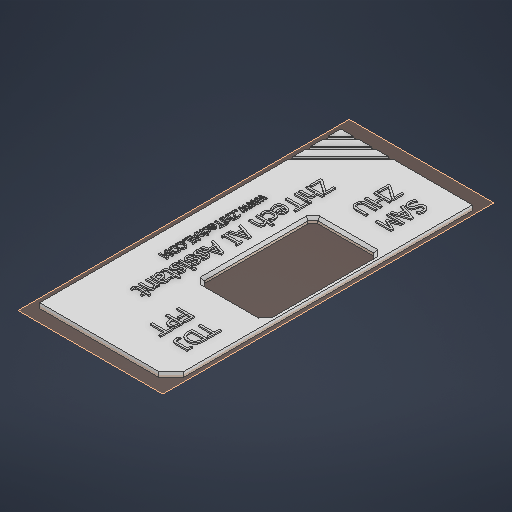
# Autodesk Inventor part: Part6
Saved by Autodesk Inventor 2026 (Build 300175000, 175)
## iProperties
Created: 2025-06-06
Part Number: Part6
Material: Generic
Document SubType Name: Sheet Metal
Designer: ziyuz
Density: 1 g/cm^3
Sheet Metal Rule: Default_mm
Appearance: Default
Author: ziyuz
Autodesk Inventor part; units mm, degrees
(part 1 of 2)
ref_plane "YZ Plane" through (0, 0, 0) normal (1, 0, 0) x (0, 1, 0)
ref_plane "XZ Plane" through (0, 0, 0) normal (0, 1, 0) x (-1, 0, 0)
ref_plane "XY Plane" through (0, 0, 0) normal (0, 0, 1) x (1, 0, 0)
sketch "Sketch1" plane through (0, 0, 0) normal (0, 1, 0) x (-1, 0, 0)
  line L0 (-29.0932, -58.6501) -> (-29.0932, -48.6501)
  line L1 (-29.0932, -58.6501) -> (-29.0932, 55.3499)
  line L2 (-29.0932, 55.3499) -> (-24.0932, 60.3499)
  line L3 (-29.0932, 55.3499) -> (-24.0932, 60.3499)
  line L4 (-24.0932, 60.3499) -> (22.9068, 60.3499)
  line L5 (-24.0932, 60.3499) -> (22.9068, 60.3499)
  line L6 (22.9068, 60.3499) -> (22.9068, -58.6501)
  line L7 (22.9068, -58.6501) -> (-29.0932, -58.6501)
  line L8 (-29.0932, -38.6501) -> (0.9068, -38.6501)
  line L9 (-29.0932, -38.6501) -> (2.9068, -38.6501)
  line L10 (2.9068, -38.6501) -> (2.9068, 31.3499)
  line L11 (2.9068, 31.3499) -> (-29.0932, 31.3499)
  line L12 (-29.0932, -38.6501) -> (-29.0932, -23.6501)
  line L13 (-29.0932, -23.6501) -> (2.9068, -23.6501)
  line L14 (-29.0932, 31.3499) -> (-29.0932, 21.3499)
  line L15 (-29.0932, 21.3499) -> (2.9068, 21.3499)
  line L16 (-29.0932, -23.6501) -> (-29.0932, 21.3499)
  line L17 (-29.0932, -23.6501) -> (-27.0932, -23.6501)
  line L18 (-27.0932, -23.6501) -> (-27.0932, 21.3499)
  line L19 (-29.0932, 21.3499) -> (-27.0932, 21.3499)
  line L20 (0.9068, -38.6501) -> (0.9068, 31.3499)
  line L21 (0.9068, -23.6501) -> (-1.0932, -23.6501)
  line L22 (-1.0932, -23.6501) -> (-1.0932, 21.3499)
  point P0 (0, 0)
  point P1 (-27.0932, 58.3499)
  dimension "d0" = 32
  dimension "d1" = 70
  dimension "d2" = 15
  dimension "d3" = 10
  dimension "d4" = 2
  dimension "d5" = 2
  constraints: 46 end point, 11 point on line, 8 perpendicular, 5 collinear, 1 vertical
  measures "d0" distance of L8.start L9.end
  measures "d1" distance of L9.end L10.end
  measures "d2" distance of L8.start L12.end
  measures "d3" distance of L11.end L14.end
  measures "d4" distance of L12.end L17.end
  measures "d5" distance of L21.start L21.end
extrude "Extrusion1" add sketch "Sketch1" along normal blind 2 contours L0 L1 L8 L9 L10 L11 L2 L4 L6 L7 | L1 L13 L20 L8 | L1 L15 L18 L13 | L20 L13 L10 L9 | L1 L11 L20 L15 | L20 L15 L10 L13 | L13 L22 L15 L20 | L20 L11 L10 L15
chamfer "Chamfer1" distance 2 angle 45 4 edges at (27.0932, 1, 21.3499) (27.0932, 1, -23.6501) (1.0932, 1, -23.6501) (1.0932, 1, 21.3499)
ref_plane "Work Plane1" through (0, 1, 0) normal (0, 1, 0) x (1, 0, 0)
sketch "Sketch7" plane through (0, 2, 0) normal (0, 1, 0) x (1, 0, 0)
  line L0 (22.864, -34.3556) -> (22.864, -48.4389) construction
  line L1 (22.864, -48.4389) -> (6.7205, -48.4389) construction
  line L2 (6.7205, -48.4389) -> (6.7205, -34.3556) construction
  line L3 (6.7205, -34.3556) -> (22.864, -34.3556) construction
  line L4 (22.2427, 49.0186) -> (22.2427, 34.9352) construction
  line L5 (22.2427, 34.9352) -> (6.0992, 34.9352) construction
  line L6 (6.0992, 34.9352) -> (6.0992, 49.0186) construction
  line L7 (6.0992, 49.0186) -> (22.2427, 49.0186) construction
  line L8 (-2.8839, 40.5637) -> (-2.8839, -41.6354) construction
  line L9 (-2.8839, -41.6354) -> (-17.8366, -41.6354) construction
  line L10 (-17.8366, -41.6354) -> (-17.8366, 40.5637) construction
  line L11 (-17.8366, 40.5637) -> (-2.8839, 40.5637) construction
  line L12 (16.764, -36.3971) -> (22.1423, -36.3971)
  line L13 (22.1423, -36.3971) -> (22.1423, -34.3506)
  line L14 (22.1423, -34.3506) -> (22.864, -34.3506)
  line L15 (22.864, -34.3506) -> (22.864, -39.2543)
  line L16 (22.864, -39.2543) -> (22.1423, -39.2543)
  line L17 (22.1423, -39.2543) -> (22.1423, -37.2078)
  line L18 (22.1423, -37.2078) -> (16.764, -37.2078)
  line L19 (16.764, -37.2078) -> (16.764, -36.3971)
  spline S0 degree 2 poles (19.8091, -44.6821) (18.9737, -44.6821) (17.6291, -44.0048) (17.2534, -43.4363) knots 0 0 0 1 2 2 2
  spline S1 degree 2 poles (17.2534, -43.4363) (16.9617, -42.9717) (16.764, -42.0176) (16.764, -41.2761) knots 0 0 0 1 2 2 2
  line L20 (16.764, -41.2761) -> (16.764, -39.8722)
  line L21 (16.764, -39.8722) -> (22.864, -39.8722)
  line L22 (22.864, -39.8722) -> (22.864, -41.2613)
  spline S2 degree 2 poles (22.864, -41.2613) (22.864, -42.1214) (22.607, -43.1002) (22.3796, -43.4462) knots 0 0 0 1 2 2 2
  spline S3 degree 2 poles (22.3796, -43.4462) (21.989, -44.0345) (20.6989, -44.6821) (19.8091, -44.6821) knots 0 0 0 1 2 2 2
  spline S4 degree 2 poles (19.819, -43.8368) (20.5209, -43.8368) (21.5145, -43.3721) (21.7963, -42.9124) knots 0 0 0 1 2 2 2
  spline S5 degree 2 poles (21.7963, -42.9124) (21.989, -42.5861) (22.1621, -41.8496) (22.1621, -41.3009) knots 0 0 0 1 2 2 2
  line L23 (22.1621, -41.3009) -> (22.1621, -40.6829)
  line L24 (22.1621, -40.6829) -> (17.466, -40.6829)
  line L25 (17.466, -40.6829) -> (17.466, -41.3009)
  spline S6 degree 2 poles (17.466, -41.3009) (17.466, -41.8397) (17.639, -42.6553) (17.8713, -42.9865) knots 0 0 0 1 2 2 2
  spline S7 degree 2 poles (17.8713, -42.9865) (18.158, -43.4116) (19.1071, -43.8368) (19.819, -43.8368) knots 0 0 0 1 2 2 2
  spline S8 degree 2 poles (18.3508, -47.8606) (17.55, -47.8606) (16.68, -46.8818) (16.68, -46.0563) knots 0 0 0 1 2 2 2
  spline S9 degree 2 poles (16.68, -46.0563) (16.68, -45.8586) (16.7492, -45.2011) (16.7986, -44.9787) knots 0 0 0 1 2 2 2
  line L26 (16.7986, -44.9787) -> (17.5796, -44.9787)
  line L27 (17.5796, -44.9787) -> (17.5796, -45.0231)
  spline S10 degree 2 poles (17.5796, -45.0231) (17.5203, -45.1912) (17.3819, -45.6905) (17.3819, -45.9475) knots 0 0 0 1 2 2 2
  spline S11 degree 2 poles (17.3819, -45.9475) (17.3819, -46.3232) (17.5549, -46.7731) (17.7131, -46.8769) knots 0 0 0 1 2 2 2
  spline S12 degree 2 poles (17.7131, -46.8769) (17.8762, -46.9906) (18.3508, -47.0499) (18.6622, -47.0499) knots 0 0 0 1 2 2 2
  line L28 (18.6622, -47.0499) -> (22.2164, -47.0499)
  line L29 (22.2164, -47.0499) -> (22.2164, -45.7597)
  line L30 (22.2164, -45.7597) -> (22.864, -45.7597)
  line L31 (22.864, -45.7597) -> (22.864, -47.8606)
  line L32 (22.864, -47.8606) -> (18.3508, -47.8606)
  line L33 (12.0988, -38.6216) -> (12.0988, -35.7842)
  line L34 (12.0988, -35.7842) -> (10.3785, -35.7842)
  line L35 (10.3785, -35.7842) -> (10.3785, -38.503)
  line L36 (10.3785, -38.503) -> (9.6568, -38.503)
  line L37 (9.6568, -38.503) -> (9.6568, -35.7842)
  line L38 (9.6568, -35.7842) -> (6.7205, -35.7842)
  line L39 (6.7205, -35.7842) -> (6.7205, -34.9735)
  line L40 (6.7205, -34.9735) -> (12.8205, -34.9735)
  line L41 (12.8205, -34.9735) -> (12.8205, -38.6216)
  line L42 (12.8205, -38.6216) -> (12.0988, -38.6216)
  spline S13 degree 2 poles (10.9816, -43.204) (10.5862, -43.204) (9.8743, -42.9222) (9.6272, -42.6701) knots 0 0 0 1 2 2 2
  spline S14 degree 2 poles (9.6272, -42.6701) (9.3157, -42.3538) (8.9944, -41.4986) (8.9944, -40.8461) knots 0 0 0 1 2 2 2
  line L43 (8.9944, -40.8461) -> (8.9944, -40.159)
  line L44 (8.9944, -40.159) -> (6.7205, -40.159)
  line L45 (6.7205, -40.159) -> (6.7205, -39.3483)
  line L46 (6.7205, -39.3483) -> (12.8205, -39.3483)
  line L47 (12.8205, -39.3483) -> (12.8205, -40.8807)
  spline S15 degree 2 poles (12.8205, -40.8807) (12.8205, -41.4244) (12.6426, -42.1857) (12.4399, -42.4774) knots 0 0 0 1 2 2 2
  spline S16 degree 2 poles (12.4399, -42.4774) (12.2076, -42.8184) (11.4908, -43.204) (10.9816, -43.204) knots 0 0 0 1 2 2 2
  spline S17 degree 2 poles (10.9569, -42.3587) (11.2733, -42.3587) (11.7379, -42.1412) (11.8862, -41.9188) knots 0 0 0 1 2 2 2
  spline S18 degree 2 poles (11.8862, -41.9188) (12.0148, -41.726) (12.1186, -41.2119) (12.1186, -40.8312) knots 0 0 0 1 2 2 2
  line L48 (12.1186, -40.8312) -> (12.1186, -40.159)
  line L49 (12.1186, -40.159) -> (9.6865, -40.159)
  line L50 (9.6865, -40.159) -> (9.6865, -40.7126)
  spline S19 degree 2 poles (9.6865, -40.7126) (9.6865, -41.2069) (9.8447, -41.815) (10.0523, -42.0127) knots 0 0 0 1 2 2 2
  spline S20 degree 2 poles (10.0523, -42.0127) (10.2352, -42.1956) (10.6653, -42.3587) (10.9569, -42.3587) knots 0 0 0 1 2 2 2
  line L51 (6.7205, -45.3988) -> (12.0988, -45.3988)
  line L52 (12.0988, -45.3988) -> (12.0988, -43.3523)
  line L53 (12.0988, -43.3523) -> (12.8205, -43.3523)
  line L54 (12.8205, -43.3523) -> (12.8205, -48.256)
  line L55 (12.8205, -48.256) -> (12.0988, -48.256)
  line L56 (12.0988, -48.256) -> (12.0988, -46.2095)
  line L57 (12.0988, -46.2095) -> (6.7205, -46.2095)
  line L58 (6.7205, -46.2095) -> (6.7205, -45.3988)
  point P0 (0, 0)
  constraints: 6 other
extrude "Extrusion6" add sketch "Sketch7" along normal blind 0.5
sketch "Sketch8" plane through (0, 2, 0) normal (0, 1, 0) x (1, 0, 0)
  line L0 (22.2544, 48.9464) -> (22.2544, 32.777) construction
  line L1 (22.2544, 32.777) -> (5.8736, 32.777) construction
  line L2 (5.8736, 32.777) -> (5.8736, 48.9464) construction
  line L3 (5.8736, 48.9464) -> (22.2544, 48.9464) construction
  spline S0 degree 2 poles (15.9369, 46.628) (15.9369, 47.2904) (16.2137, 48.2197) (16.4114, 48.63) knots 0 0 0 1 2 2 2
  line L4 (16.4114, 48.63) -> (17.4297, 48.63)
  line L5 (17.4297, 48.63) -> (17.4297, 48.5707)
  spline S1 degree 2 poles (17.4297, 48.5707) (17.054, 48.1703) (16.6388, 47.1569) (16.6388, 46.6873) knots 0 0 0 1 2 2 2
  spline S2 degree 2 poles (16.6388, 46.6873) (16.6388, 46.015) (17.1974, 45.3279) (17.6571, 45.3279) knots 0 0 0 1 2 2 2
  spline S3 degree 2 poles (17.6571, 45.3279) (18.0229, 45.3279) (18.4777, 45.6888) (18.5914, 46.0793) knots 0 0 0 1 2 2 2
  spline S4 degree 2 poles (18.5914, 46.0793) (18.6705, 46.3611) (18.7792, 46.8307) (18.8682, 47.1817) knots 0 0 0 1 2 2 2
  spline S5 degree 2 poles (18.8682, 47.1817) (18.9523, 47.498) (19.2044, 47.9973) (19.407, 48.1901) knots 0 0 0 1 2 2 2
  spline S6 degree 2 poles (19.407, 48.1901) (19.6097, 48.3779) (20.1535, 48.5856) (20.5094, 48.5856) knots 0 0 0 1 2 2 2
  spline S7 degree 2 poles (20.5094, 48.5856) (21.2509, 48.5856) (22.2544, 47.4288) (22.2544, 46.5341) knots 0 0 0 1 2 2 2
  spline S8 degree 2 poles (22.2544, 46.5341) (22.2544, 46.02) (22.0517, 45.1104) (21.8589, 44.7199) knots 0 0 0 1 2 2 2
  line L6 (21.8589, 44.7199) -> (20.89, 44.7199)
  line L7 (20.89, 44.7199) -> (20.89, 44.7792)
  spline S9 degree 2 poles (20.89, 44.7792) (21.157, 45.0709) (21.5524, 45.9804) (21.5524, 46.4797) knots 0 0 0 1 2 2 2
  spline S10 degree 2 poles (21.5524, 46.4797) (21.5524, 47.0433) (21.0235, 47.7403) (20.5934, 47.7403) knots 0 0 0 1 2 2 2
  spline S11 degree 2 poles (20.5934, 47.7403) (20.2079, 47.7403) (19.7481, 47.33) (19.6443, 46.9444) knots 0 0 0 1 2 2 2
  spline S12 degree 2 poles (19.6443, 46.9444) (19.5751, 46.6873) (19.3972, 45.9409) (19.323, 45.6937) knots 0 0 0 1 2 2 2
  spline S13 degree 2 poles (19.323, 45.6937) (19.1302, 45.0659) (18.3541, 44.4826) (17.7856, 44.4826) knots 0 0 0 1 2 2 2
  spline S14 degree 2 poles (17.7856, 44.4826) (17.4248, 44.4826) (16.7327, 44.7743) (16.4905, 45.0363) knots 0 0 0 1 2 2 2
  spline S15 degree 2 poles (16.4905, 45.0363) (16.2236, 45.3279) (15.9369, 46.0694) (15.9369, 46.628) knots 0 0 0 1 2 2 2
  line L8 (16.0456, 44.3146) -> (22.1456, 42.2582)
  line L9 (22.1456, 42.2582) -> (22.1456, 41.2596)
  line L10 (22.1456, 41.2596) -> (16.0456, 39.2032)
  line L11 (16.0456, 39.2032) -> (16.0456, 40.0584)
  line L12 (16.0456, 40.0584) -> (17.751, 40.6121)
  line L13 (17.751, 40.6121) -> (17.751, 42.9403)
  line L14 (17.751, 42.9403) -> (16.0456, 43.494)
  line L15 (16.0456, 43.494) -> (16.0456, 44.3146)
  line L16 (18.4431, 40.8345) -> (21.3151, 41.7787)
  line L17 (21.3151, 41.7787) -> (18.4431, 42.7179)
  line L18 (18.4431, 42.7179) -> (18.4431, 40.8345)
  line L19 (16.0456, 33.3949) -> (16.0456, 34.2056)
  line L20 (16.0456, 34.2056) -> (21.3003, 34.2056)
  line L21 (21.3003, 34.2056) -> (17.7263, 35.7973)
  line L22 (17.7263, 35.7973) -> (17.7263, 36.2916)
  line L23 (17.7263, 36.2916) -> (21.3003, 37.8685)
  line L24 (21.3003, 37.8685) -> (16.0456, 37.8685)
  line L25 (16.0456, 37.8685) -> (16.0456, 38.6249)
  line L26 (16.0456, 38.6249) -> (22.1456, 38.6249)
  line L27 (22.1456, 38.6249) -> (22.1456, 37.5176)
  line L28 (22.1456, 37.5176) -> (18.7496, 35.995)
  line L29 (18.7496, 35.995) -> (22.1456, 34.5219)
  line L30 (22.1456, 34.5219) -> (22.1456, 33.3949)
  line L31 (22.1456, 33.3949) -> (16.0456, 33.3949)
  line L32 (6.0021, 44.4381) -> (6.0021, 48.6992)
  line L33 (6.0021, 48.6992) -> (6.7584, 48.6992)
  line L34 (6.7584, 48.6992) -> (11.3804, 45.4367)
  line L35 (11.3804, 45.4367) -> (11.3804, 48.5509)
  line L36 (11.3804, 48.5509) -> (12.1021, 48.5509)
  line L37 (12.1021, 48.5509) -> (12.1021, 44.5222)
  line L38 (12.1021, 44.5222) -> (11.3705, 44.5222)
  line L39 (11.3705, 44.5222) -> (6.7238, 47.8193)
  line L40 (6.7238, 47.8193) -> (6.7238, 44.4381)
  line L41 (6.7238, 44.4381) -> (6.0021, 44.4381)
  line L42 (6.0021, 39.2082) -> (6.0021, 40.0189)
  line L43 (6.0021, 40.0189) -> (8.9879, 40.0189)
  line L44 (8.9879, 40.0189) -> (8.9879, 42.8266)
  line L45 (8.9879, 42.8266) -> (6.0021, 42.8266)
  line L46 (6.0021, 42.8266) -> (6.0021, 43.6373)
  line L47 (6.0021, 43.6373) -> (12.1021, 43.6373)
  line L48 (12.1021, 43.6373) -> (12.1021, 42.8266)
  line L49 (12.1021, 42.8266) -> (9.7096, 42.8266)
  line L50 (9.7096, 42.8266) -> (9.7096, 40.0189)
  line L51 (9.7096, 40.0189) -> (12.1021, 40.0189)
  line L52 (12.1021, 40.0189) -> (12.1021, 39.2082)
  line L53 (12.1021, 39.2082) -> (6.0021, 39.2082)
  spline S16 degree 2 poles (5.8736, 35.8418) (5.8736, 36.3806) (6.1554, 37.1814) (6.4371, 37.4632) knots 0 0 0 1 2 2 2
  spline S17 degree 2 poles (6.4371, 37.4632) (6.7535, 37.7845) (7.6433, 38.0465) (8.2958, 38.0465) knots 0 0 0 1 2 2 2
  line L54 (8.2958, 38.0465) -> (12.1021, 38.0465)
  line L55 (12.1021, 38.0465) -> (12.1021, 37.2358)
  line L56 (12.1021, 37.2358) -> (8.2958, 37.2358)
  spline S18 degree 2 poles (8.2958, 37.2358) (7.8707, 37.2358) (7.2973, 37.127) (7.0649, 36.9738) knots 0 0 0 1 2 2 2
  spline S19 degree 2 poles (7.0649, 36.9738) (6.8178, 36.8107) (6.5657, 36.2471) (6.5657, 35.8418) knots 0 0 0 1 2 2 2
  spline S20 degree 2 poles (6.5657, 35.8418) (6.5657, 35.4612) (6.8178, 34.868) (7.0649, 34.7048) knots 0 0 0 1 2 2 2
  spline S21 degree 2 poles (7.0649, 34.7048) (7.2973, 34.5516) (7.8657, 34.4428) (8.276, 34.4428) knots 0 0 0 1 2 2 2
  line L57 (8.276, 34.4428) -> (12.1021, 34.4428)
  line L58 (12.1021, 34.4428) -> (12.1021, 33.6321)
  line L59 (12.1021, 33.6321) -> (8.2958, 33.6321)
  spline S22 degree 2 poles (8.2958, 33.6321) (7.6581, 33.6321) (6.7486, 33.8892) (6.4371, 34.2155) knots 0 0 0 1 2 2 2
  spline S23 degree 2 poles (6.4371, 34.2155) (6.1504, 34.5071) (5.8736, 35.2783) (5.8736, 35.8418) knots 0 0 0 1 2 2 2
  point P0 (0, 0)
  constraints: 2 other
extrude "Extrusion7" add sketch "Sketch8" along normal blind 0.5
sketch "Sketch9" plane through (0, 2, 0) normal (0, 1, 0) x (1, 0, 0)
  line L0 (-3.0335, 37.4291) -> (-3.0335, -37.9904) construction
  line L1 (-3.0335, -37.9904) -> (-36.9755, -37.9904) construction
  line L2 (-36.9755, -37.9904) -> (-36.9755, 37.4291) construction
  line L3 (-36.9755, 37.4291) -> (-3.0335, 37.4291) construction
  line L4 (-9.4054, 32.9209) -> (-9.4054, 37.182)
  line L5 (-9.4054, 37.182) -> (-8.6491, 37.182)
  line L6 (-8.6491, 37.182) -> (-4.0271, 33.9194)
  line L7 (-4.0271, 33.9194) -> (-4.0271, 37.0337)
  line L8 (-4.0271, 37.0337) -> (-3.3054, 37.0337)
  line L9 (-3.3054, 37.0337) -> (-3.3054, 33.0049)
  line L10 (-3.3054, 33.0049) -> (-4.037, 33.0049)
  line L11 (-4.037, 33.0049) -> (-8.6837, 36.3021)
  line L12 (-8.6837, 36.3021) -> (-8.6837, 32.9209)
  line L13 (-8.6837, 32.9209) -> (-9.4054, 32.9209)
  line L14 (-9.4054, 28.5856) -> (-9.4054, 29.3568)
  line L15 (-9.4054, 29.3568) -> (-6.7954, 29.3568)
  spline S0 degree 2 poles (-6.7954, 29.3568) (-6.479, 29.3568) (-5.9352, 29.4161) (-5.7721, 29.5051) knots 0 0 0 1 2 2 2
  spline S1 degree 2 poles (-5.7721, 29.5051) (-5.5991, 29.599) (-5.431, 29.9351) (-5.431, 30.2218) knots 0 0 0 1 2 2 2
  spline S2 degree 2 poles (-5.431, 30.2218) (-5.431, 30.5086) (-5.7375, 31.1166) (-5.9847, 31.4082) knots 0 0 0 1 2 2 2
  line L16 (-5.9847, 31.4082) -> (-9.4054, 31.4082)
  line L17 (-9.4054, 31.4082) -> (-9.4054, 32.1794)
  line L18 (-9.4054, 32.1794) -> (-3.0335, 32.1794)
  line L19 (-3.0335, 32.1794) -> (-3.0335, 31.4082)
  line L20 (-3.0335, 31.4082) -> (-5.3371, 31.4082)
  spline S3 degree 2 poles (-5.3371, 31.4082) (-5.0257, 31.0622) (-4.6994, 30.3949) (-4.6994, 30.0192) knots 0 0 0 1 2 2 2
  spline S4 degree 2 poles (-4.6994, 30.0192) (-4.6994, 29.3469) (-5.5892, 28.5856) (-6.4345, 28.5856) knots 0 0 0 1 2 2 2
  line L21 (-6.4345, 28.5856) -> (-9.4054, 28.5856)
  line L22 (-9.4054, 26.7171) -> (-9.4054, 27.4882)
  line L23 (-9.4054, 27.4882) -> (-4.8279, 27.4882)
  line L24 (-4.8279, 27.4882) -> (-4.8279, 26.7171)
  line L25 (-4.8279, 26.7171) -> (-9.4054, 26.7171)
  line L26 (-4.0667, 26.6627) -> (-4.0667, 27.5377)
  line L27 (-4.0667, 27.5377) -> (-3.2659, 27.5377)
  line L28 (-3.2659, 27.5377) -> (-3.2659, 26.6627)
  line L29 (-3.2659, 26.6627) -> (-4.0667, 26.6627)
  line L30 (-9.4054, 24.1021) -> (-4.0271, 24.1021)
  line L31 (-4.0271, 24.1021) -> (-4.0271, 26.1486)
  line L32 (-4.0271, 26.1486) -> (-3.3054, 26.1486)
  line L33 (-3.3054, 26.1486) -> (-3.3054, 21.2449)
  line L34 (-3.3054, 21.2449) -> (-4.0271, 21.2449)
  line L35 (-4.0271, 21.2449) -> (-4.0271, 23.2914)
  line L36 (-4.0271, 23.2914) -> (-9.4054, 23.2914)
  line L37 (-9.4054, 23.2914) -> (-9.4054, 24.1021)
  spline S5 degree 2 poles (-9.5092, 18.6991) (-9.5092, 19.7965) (-8.2783, 21.0026) (-7.1414, 21.0026) knots 0 0 0 1 2 2 2
  spline S6 degree 2 poles (-7.1414, 21.0026) (-6.0242, 21.0026) (-4.6994, 19.8311) (-4.6994, 18.8869) knots 0 0 0 1 2 2 2
  spline S7 degree 2 poles (-4.6994, 18.8869) (-4.6994, 18.4618) (-4.9466, 17.8043) (-5.2086, 17.5621) knots 0 0 0 1 2 2 2
  spline S8 degree 2 poles (-5.2086, 17.5621) (-5.4706, 17.315) (-6.2269, 17.053) (-6.7756, 17.053) knots 0 0 0 1 2 2 2
  line L38 (-6.7756, 17.053) -> (-7.1958, 17.053)
  line L39 (-7.1958, 17.053) -> (-7.1958, 20.2216)
  spline S9 degree 2 poles (-7.1958, 20.2216) (-7.9916, 20.2216) (-8.8369, 19.4208) (-8.8369, 18.709) knots 0 0 0 1 2 2 2
  spline S10 degree 2 poles (-8.8369, 18.709) (-8.8369, 18.4569) (-8.7232, 17.9675) (-8.6343, 17.7697) knots 0 0 0 1 2 2 2
  spline S11 degree 2 poles (-8.6343, 17.7697) (-8.5354, 17.5621) (-8.3624, 17.2754) (-8.2833, 17.1815) knots 0 0 0 1 2 2 2
  line L40 (-8.2833, 17.1815) -> (-8.2833, 17.137)
  line L41 (-8.2833, 17.137) -> (-9.1236, 17.137)
  spline S12 degree 2 poles (-9.1236, 17.137) (-9.178, 17.2705) (-9.3362, 17.6758) (-9.3807, 17.834) knots 0 0 0 1 2 2 2
  spline S13 degree 2 poles (-9.3807, 17.834) (-9.445, 18.0565) (-9.5092, 18.4223) (-9.5092, 18.6991) knots 0 0 0 1 2 2 2
  spline S14 degree 2 poles (-6.6075, 17.8043) (-6.2961, 17.8142) (-5.8413, 17.9428) (-5.6881, 18.0663) knots 0 0 0 1 2 2 2
  spline S15 degree 2 poles (-5.6881, 18.0663) (-5.5151, 18.1998) (-5.3321, 18.62) (-5.3321, 18.9314) knots 0 0 0 1 2 2 2
  spline S16 degree 2 poles (-5.3321, 18.9314) (-5.3321, 19.2379) (-5.5151, 19.668) (-5.693, 19.8459) knots 0 0 0 1 2 2 2
  spline S17 degree 2 poles (-5.693, 19.8459) (-5.8759, 20.0189) (-6.3159, 20.1969) (-6.6075, 20.2216) knots 0 0 0 1 2 2 2
  line L42 (-6.6075, 20.2216) -> (-6.6075, 17.8043)
  spline S18 degree 2 poles (-9.5092, 14.4528) (-9.5092, 14.9274) (-9.2176, 15.7133) (-8.921, 15.9951) knots 0 0 0 1 2 2 2
  spline S19 degree 2 poles (-8.921, 15.9951) (-8.6293, 16.2769) (-7.7296, 16.5883) (-7.1266, 16.5883) knots 0 0 0 1 2 2 2
  spline S20 degree 2 poles (-7.1266, 16.5883) (-6.5235, 16.5883) (-5.6436, 16.267) (-5.347, 15.9951) knots 0 0 0 1 2 2 2
  spline S21 degree 2 poles (-5.347, 15.9951) (-5.0454, 15.7232) (-4.7241, 14.9175) (-4.7241, 14.4528) knots 0 0 0 1 2 2 2
  spline S22 degree 2 poles (-4.7241, 14.4528) (-4.7241, 14.0771) (-4.9367, 13.3752) (-5.0751, 13.1033) knots 0 0 0 1 2 2 2
  line L43 (-5.0751, 13.1033) -> (-5.9402, 13.1033)
  line L44 (-5.9402, 13.1033) -> (-5.9402, 13.1478)
  spline S23 degree 2 poles (-5.9402, 13.1478) (-5.871, 13.2318) (-5.693, 13.4889) (-5.5991, 13.6718) knots 0 0 0 1 2 2 2
  spline S24 degree 2 poles (-5.5991, 13.6718) (-5.52, 13.8349) (-5.3964, 14.2699) (-5.3964, 14.4676) knots 0 0 0 1 2 2 2
  spline S25 degree 2 poles (-5.3964, 14.4676) (-5.3964, 15.0658) (-6.301, 15.7924) (-7.1266, 15.7924) knots 0 0 0 1 2 2 2
  spline S26 degree 2 poles (-7.1266, 15.7924) (-7.9323, 15.7924) (-8.8369, 15.0905) (-8.8369, 14.4676) knots 0 0 0 1 2 2 2
  spline S27 degree 2 poles (-8.8369, 14.4676) (-8.8369, 14.0919) (-8.5255, 13.4098) (-8.2833, 13.1478) knots 0 0 0 1 2 2 2
  line L45 (-8.2833, 13.1478) -> (-8.2833, 13.1033)
  line L46 (-8.2833, 13.1033) -> (-9.1484, 13.1033)
  spline S28 degree 2 poles (-9.1484, 13.1033) (-9.2027, 13.217) (-9.356, 13.563) (-9.3906, 13.7014) knots 0 0 0 1 2 2 2
  spline S29 degree 2 poles (-9.3906, 13.7014) (-9.4499, 13.8992) (-9.5092, 14.2106) (-9.5092, 14.4528) knots 0 0 0 1 2 2 2
  line L47 (-9.4054, 8.8076) -> (-9.4054, 9.5787)
  line L48 (-9.4054, 9.5787) -> (-6.7954, 9.5787)
  spline S30 degree 2 poles (-6.7954, 9.5787) (-6.479, 9.5787) (-5.9352, 9.6381) (-5.7721, 9.727) knots 0 0 0 1 2 2 2
  spline S31 degree 2 poles (-5.7721, 9.727) (-5.5991, 9.821) (-5.431, 10.1571) (-5.431, 10.4438) knots 0 0 0 1 2 2 2
  spline S32 degree 2 poles (-5.431, 10.4438) (-5.431, 10.7305) (-5.7375, 11.3385) (-5.9847, 11.6302) knots 0 0 0 1 2 2 2
  line L49 (-5.9847, 11.6302) -> (-9.4054, 11.6302)
  line L50 (-9.4054, 11.6302) -> (-9.4054, 12.4013)
  line L51 (-9.4054, 12.4013) -> (-3.0335, 12.4013)
  line L52 (-3.0335, 12.4013) -> (-3.0335, 11.6302)
  line L53 (-3.0335, 11.6302) -> (-5.3371, 11.6302)
  spline S33 degree 2 poles (-5.3371, 11.6302) (-5.0257, 11.2842) (-4.6994, 10.6168) (-4.6994, 10.2411) knots 0 0 0 1 2 2 2
  spline S34 degree 2 poles (-4.6994, 10.2411) (-4.6994, 9.5689) (-5.5892, 8.8076) (-6.4345, 8.8076) knots 0 0 0 1 2 2 2
  line L54 (-6.4345, 8.8076) -> (-9.4054, 8.8076)
  line L55 (-9.4054, 5.7032) -> (-3.3054, 3.6468)
  line L56 (-3.3054, 3.6468) -> (-3.3054, 2.6483)
  line L57 (-3.3054, 2.6483) -> (-9.4054, 0.5919)
  line L58 (-9.4054, 0.5919) -> (-9.4054, 1.4471)
  line L59 (-9.4054, 1.4471) -> (-7.7, 2.0007)
  line L60 (-7.7, 2.0007) -> (-7.7, 4.329)
  line L61 (-7.7, 4.329) -> (-9.4054, 4.8826)
  line L62 (-9.4054, 4.8826) -> (-9.4054, 5.7032)
  line L63 (-7.0079, 2.2231) -> (-4.1359, 3.1673)
  line L64 (-4.1359, 3.1673) -> (-7.0079, 4.1065)
  line L65 (-7.0079, 4.1065) -> (-7.0079, 2.2231)
  line L66 (-9.4054, -2.1121) -> (-9.4054, 0.2508)
  line L67 (-9.4054, 0.2508) -> (-8.7826, 0.2508)
  line L68 (-8.7826, 0.2508) -> (-8.7826, -0.5253)
  line L69 (-8.7826, -0.5253) -> (-3.9283, -0.5253)
  line L70 (-3.9283, -0.5253) -> (-3.9283, 0.2508)
  line L71 (-3.9283, 0.2508) -> (-3.3054, 0.2508)
  line L72 (-3.3054, 0.2508) -> (-3.3054, -2.1121)
  line L73 (-3.3054, -2.1121) -> (-3.9283, -2.1121)
  line L74 (-3.9283, -2.1121) -> (-3.9283, -1.336)
  line L75 (-3.9283, -1.336) -> (-8.7826, -1.336)
  line L76 (-8.7826, -1.336) -> (-8.7826, -2.1121)
  line L77 (-8.7826, -2.1121) -> (-9.4054, -2.1121)
  line L78 (-9.4054, -5.0781) -> (-3.3054, -7.1345)
  line L79 (-3.3054, -7.1345) -> (-3.3054, -8.133)
  line L80 (-3.3054, -8.133) -> (-9.4054, -10.1894)
  line L81 (-9.4054, -10.1894) -> (-9.4054, -9.3342)
  line L82 (-9.4054, -9.3342) -> (-7.7, -8.7806)
  line L83 (-7.7, -8.7806) -> (-7.7, -6.4523)
  line L84 (-7.7, -6.4523) -> (-9.4054, -5.8987)
  line L85 (-9.4054, -5.8987) -> (-9.4054, -5.0781)
  line L86 (-7.0079, -8.5581) -> (-4.1359, -7.614)
  line L87 (-4.1359, -7.614) -> (-7.0079, -6.6747)
  line L88 (-7.0079, -6.6747) -> (-7.0079, -8.5581)
  spline S35 degree 2 poles (-9.5142, -11.9443) (-9.5142, -11.4846) (-9.267, -10.6887) (-9.1286, -10.4267) knots 0 0 0 1 2 2 2
  line L89 (-9.1286, -10.4267) -> (-8.2635, -10.4267)
  line L90 (-8.2635, -10.4267) -> (-8.2635, -10.4662)
  spline S36 degree 2 poles (-8.2635, -10.4662) (-8.3426, -10.5651) (-8.5304, -10.832) (-8.6343, -11.0545) knots 0 0 0 1 2 2 2
  spline S37 degree 2 poles (-8.6343, -11.0545) (-8.7282, -11.2473) (-8.8666, -11.7218) (-8.8666, -11.9739) knots 0 0 0 1 2 2 2
  spline S38 degree 2 poles (-8.8666, -11.9739) (-8.8666, -12.1568) (-8.7826, -12.577) (-8.7133, -12.6759) knots 0 0 0 1 2 2 2
  spline S39 degree 2 poles (-8.7133, -12.6759) (-8.6194, -12.8192) (-8.4069, -12.9478) (-8.1894, -12.9478) knots 0 0 0 1 2 2 2
  spline S40 degree 2 poles (-8.1894, -12.9478) (-7.9175, -12.9478) (-7.6357, -12.6512) (-7.5418, -12.2705) knots 0 0 0 1 2 2 2
  spline S41 degree 2 poles (-7.5418, -12.2705) (-7.5072, -12.1222) (-7.4083, -11.6477) (-7.3539, -11.445) knots 0 0 0 1 2 2 2
  spline S42 degree 2 poles (-7.3539, -11.445) (-7.2007, -10.921) (-6.568, -10.4465) (-6.1181, -10.4465) knots 0 0 0 1 2 2 2
  spline S43 degree 2 poles (-6.1181, -10.4465) (-5.4953, -10.4465) (-4.7192, -11.3807) (-4.7192, -12.1519) knots 0 0 0 1 2 2 2
  spline S44 degree 2 poles (-4.7192, -12.1519) (-4.7192, -12.5325) (-4.907, -13.3037) (-5.0504, -13.5657) knots 0 0 0 1 2 2 2
  line L91 (-5.0504, -13.5657) -> (-5.8759, -13.5657)
  line L92 (-5.8759, -13.5657) -> (-5.8759, -13.5261)
  spline S45 degree 2 poles (-5.8759, -13.5261) (-5.6386, -13.2295) (-5.3668, -12.5078) (-5.3668, -12.1371) knots 0 0 0 1 2 2 2
  spline S46 degree 2 poles (-5.3668, -12.1371) (-5.3668, -11.7564) (-5.6881, -11.2324) (-6.0094, -11.2324) knots 0 0 0 1 2 2 2
  spline S47 degree 2 poles (-6.0094, -11.2324) (-6.301, -11.2324) (-6.5828, -11.5439) (-6.6718, -11.8899) knots 0 0 0 1 2 2 2
  spline S48 degree 2 poles (-6.6718, -11.8899) (-6.7163, -12.058) (-6.8052, -12.4831) (-6.8596, -12.7154) knots 0 0 0 1 2 2 2
  spline S49 degree 2 poles (-6.8596, -12.7154) (-6.9881, -13.2196) (-7.5764, -13.7337) (-8.0856, -13.7337) knots 0 0 0 1 2 2 2
  spline S50 degree 2 poles (-8.0856, -13.7337) (-8.3821, -13.7337) (-8.9061, -13.5014) (-9.0989, -13.274) knots 0 0 0 1 2 2 2
  spline S51 degree 2 poles (-9.0989, -13.274) (-9.3016, -13.0318) (-9.5142, -12.4139) (-9.5142, -11.9443) knots 0 0 0 1 2 2 2
  spline S52 degree 2 poles (-9.5142, -15.6863) (-9.5142, -15.2266) (-9.267, -14.4307) (-9.1286, -14.1688) knots 0 0 0 1 2 2 2
  line L93 (-9.1286, -14.1688) -> (-8.2635, -14.1688)
  line L94 (-8.2635, -14.1688) -> (-8.2635, -14.2083)
  spline S53 degree 2 poles (-8.2635, -14.2083) (-8.3426, -14.3072) (-8.5304, -14.5741) (-8.6343, -14.7965) knots 0 0 0 1 2 2 2
  spline S54 degree 2 poles (-8.6343, -14.7965) (-8.7282, -14.9893) (-8.8666, -15.4639) (-8.8666, -15.716) knots 0 0 0 1 2 2 2
  spline S55 degree 2 poles (-8.8666, -15.716) (-8.8666, -15.8989) (-8.7826, -16.3191) (-8.7133, -16.4179) knots 0 0 0 1 2 2 2
  spline S56 degree 2 poles (-8.7133, -16.4179) (-8.6194, -16.5613) (-8.4069, -16.6898) (-8.1894, -16.6898) knots 0 0 0 1 2 2 2
  spline S57 degree 2 poles (-8.1894, -16.6898) (-7.9175, -16.6898) (-7.6357, -16.3932) (-7.5418, -16.0126) knots 0 0 0 1 2 2 2
  spline S58 degree 2 poles (-7.5418, -16.0126) (-7.5072, -15.8643) (-7.4083, -15.3897) (-7.3539, -15.1871) knots 0 0 0 1 2 2 2
  spline S59 degree 2 poles (-7.3539, -15.1871) (-7.2007, -14.6631) (-6.568, -14.1885) (-6.1181, -14.1885) knots 0 0 0 1 2 2 2
  spline S60 degree 2 poles (-6.1181, -14.1885) (-5.4953, -14.1885) (-4.7192, -15.1228) (-4.7192, -15.894) knots 0 0 0 1 2 2 2
  spline S61 degree 2 poles (-4.7192, -15.894) (-4.7192, -16.2746) (-4.907, -17.0457) (-5.0504, -17.3077) knots 0 0 0 1 2 2 2
  line L95 (-5.0504, -17.3077) -> (-5.8759, -17.3077)
  line L96 (-5.8759, -17.3077) -> (-5.8759, -17.2682)
  spline S62 degree 2 poles (-5.8759, -17.2682) (-5.6386, -16.9716) (-5.3668, -16.2499) (-5.3668, -15.8791) knots 0 0 0 1 2 2 2
  spline S63 degree 2 poles (-5.3668, -15.8791) (-5.3668, -15.4985) (-5.6881, -14.9745) (-6.0094, -14.9745) knots 0 0 0 1 2 2 2
  spline S64 degree 2 poles (-6.0094, -14.9745) (-6.301, -14.9745) (-6.5828, -15.2859) (-6.6718, -15.632) knots 0 0 0 1 2 2 2
  spline S65 degree 2 poles (-6.6718, -15.632) (-6.7163, -15.8) (-6.8052, -16.2252) (-6.8596, -16.4575) knots 0 0 0 1 2 2 2
  spline S66 degree 2 poles (-6.8596, -16.4575) (-6.9881, -16.9617) (-7.5764, -17.4758) (-8.0856, -17.4758) knots 0 0 0 1 2 2 2
  spline S67 degree 2 poles (-8.0856, -17.4758) (-8.3821, -17.4758) (-8.9061, -17.2435) (-9.0989, -17.0161) knots 0 0 0 1 2 2 2
  spline S68 degree 2 poles (-9.0989, -17.0161) (-9.3016, -16.7739) (-9.5142, -16.1559) (-9.5142, -15.6863) knots 0 0 0 1 2 2 2
  line L97 (-9.4054, -18.9786) -> (-9.4054, -18.2074)
  line L98 (-9.4054, -18.2074) -> (-4.8279, -18.2074)
  line L99 (-4.8279, -18.2074) -> (-4.8279, -18.9786)
  line L100 (-4.8279, -18.9786) -> (-9.4054, -18.9786)
  line L101 (-4.0667, -19.0329) -> (-4.0667, -18.158)
  line L102 (-4.0667, -18.158) -> (-3.2659, -18.158)
  line L103 (-3.2659, -18.158) -> (-3.2659, -19.0329)
  line L104 (-3.2659, -19.0329) -> (-4.0667, -19.0329)
  spline S69 degree 2 poles (-9.5142, -21.3464) (-9.5142, -20.8867) (-9.267, -20.0908) (-9.1286, -19.8288) knots 0 0 0 1 2 2 2
  line L105 (-9.1286, -19.8288) -> (-8.2635, -19.8288)
  line L106 (-8.2635, -19.8288) -> (-8.2635, -19.8683)
  spline S70 degree 2 poles (-8.2635, -19.8683) (-8.3426, -19.9672) (-8.5304, -20.2341) (-8.6343, -20.4566) knots 0 0 0 1 2 2 2
  spline S71 degree 2 poles (-8.6343, -20.4566) (-8.7282, -20.6494) (-8.8666, -21.1239) (-8.8666, -21.376) knots 0 0 0 1 2 2 2
  spline S72 degree 2 poles (-8.8666, -21.376) (-8.8666, -21.5589) (-8.7826, -21.9791) (-8.7133, -22.078) knots 0 0 0 1 2 2 2
  spline S73 degree 2 poles (-8.7133, -22.078) (-8.6194, -22.2213) (-8.4069, -22.3499) (-8.1894, -22.3499) knots 0 0 0 1 2 2 2
  spline S74 degree 2 poles (-8.1894, -22.3499) (-7.9175, -22.3499) (-7.6357, -22.0533) (-7.5418, -21.6726) knots 0 0 0 1 2 2 2
  spline S75 degree 2 poles (-7.5418, -21.6726) (-7.5072, -21.5243) (-7.4083, -21.0498) (-7.3539, -20.8471) knots 0 0 0 1 2 2 2
  spline S76 degree 2 poles (-7.3539, -20.8471) (-7.2007, -20.3231) (-6.568, -19.8486) (-6.1181, -19.8486) knots 0 0 0 1 2 2 2
  spline S77 degree 2 poles (-6.1181, -19.8486) (-5.4953, -19.8486) (-4.7192, -20.7829) (-4.7192, -21.554) knots 0 0 0 1 2 2 2
  spline S78 degree 2 poles (-4.7192, -21.554) (-4.7192, -21.9346) (-4.907, -22.7058) (-5.0504, -22.9678) knots 0 0 0 1 2 2 2
  line L107 (-5.0504, -22.9678) -> (-5.8759, -22.9678)
  line L108 (-5.8759, -22.9678) -> (-5.8759, -22.9282)
  spline S79 degree 2 poles (-5.8759, -22.9282) (-5.6386, -22.6316) (-5.3668, -21.9099) (-5.3668, -21.5392) knots 0 0 0 1 2 2 2
  spline S80 degree 2 poles (-5.3668, -21.5392) (-5.3668, -21.1585) (-5.6881, -20.6346) (-6.0094, -20.6346) knots 0 0 0 1 2 2 2
  spline S81 degree 2 poles (-6.0094, -20.6346) (-6.301, -20.6346) (-6.5828, -20.946) (-6.6718, -21.292) knots 0 0 0 1 2 2 2
  spline S82 degree 2 poles (-6.6718, -21.292) (-6.7163, -21.4601) (-6.8052, -21.8852) (-6.8596, -22.1175) knots 0 0 0 1 2 2 2
  spline S83 degree 2 poles (-6.8596, -22.1175) (-6.9881, -22.6218) (-7.5764, -23.1359) (-8.0856, -23.1359) knots 0 0 0 1 2 2 2
  spline S84 degree 2 poles (-8.0856, -23.1359) (-8.3821, -23.1359) (-8.9061, -22.9035) (-9.0989, -22.6761) knots 0 0 0 1 2 2 2
  spline S85 degree 2 poles (-9.0989, -22.6761) (-9.3016, -22.4339) (-9.5142, -21.816) (-9.5142, -21.3464) knots 0 0 0 1 2 2 2
  spline S86 degree 2 poles (-9.4944, -25.2367) (-9.4944, -24.6089) (-8.7776, -23.9021) (-8.0015, -23.9021) knots 0 0 0 1 2 2 2
  line L109 (-8.0015, -23.9021) -> (-5.4656, -23.9021)
  line L110 (-5.4656, -23.9021) -> (-5.4656, -23.383)
  line L111 (-5.4656, -23.383) -> (-4.8279, -23.383)
  line L112 (-4.8279, -23.383) -> (-4.8279, -23.9021)
  line L113 (-4.8279, -23.9021) -> (-3.513, -23.9021)
  line L114 (-3.513, -23.9021) -> (-3.513, -24.6732)
  line L115 (-3.513, -24.6732) -> (-4.8279, -24.6732)
  line L116 (-4.8279, -24.6732) -> (-4.8279, -26.0919)
  line L117 (-4.8279, -26.0919) -> (-5.4656, -26.0919)
  line L118 (-5.4656, -26.0919) -> (-5.4656, -24.6732)
  line L119 (-5.4656, -24.6732) -> (-7.6456, -24.6732)
  spline S87 degree 2 poles (-7.6456, -24.6732) (-7.9916, -24.6732) (-8.3723, -24.6979) (-8.5354, -24.782) knots 0 0 0 1 2 2 2
  spline S88 degree 2 poles (-8.5354, -24.782) (-8.6787, -24.8512) (-8.8221, -25.1626) (-8.8221, -25.4295) knots 0 0 0 1 2 2 2
  spline S89 degree 2 poles (-8.8221, -25.4295) (-8.8221, -25.6174) (-8.7084, -25.9683) (-8.6738, -26.0474) knots 0 0 0 1 2 2 2
  line L120 (-8.6738, -26.0474) -> (-8.6738, -26.0919)
  line L121 (-8.6738, -26.0919) -> (-9.3659, -26.0919)
  spline S90 degree 2 poles (-9.3659, -26.0919) (-9.4252, -25.8744) (-9.4944, -25.4295) (-9.4944, -25.2367) knots 0 0 0 1 2 2 2
  spline S91 degree 2 poles (-8.921, -29.2111) (-8.9902, -29.1172) (-9.2373, -28.8008) (-9.3115, -28.6525) knots 0 0 0 1 2 2 2
  spline S92 degree 2 poles (-9.3115, -28.6525) (-9.4202, -28.4499) (-9.5339, -28.0692) (-9.5339, -27.7232) knots 0 0 0 1 2 2 2
  spline S93 degree 2 poles (-9.5339, -27.7232) (-9.5339, -27.4414) (-9.3214, -26.9323) (-9.1286, -26.7395) knots 0 0 0 1 2 2 2
  spline S94 degree 2 poles (-9.1286, -26.7395) (-8.9407, -26.5566) (-8.3871, -26.3341) (-8.0806, -26.3341) knots 0 0 0 1 2 2 2
  spline S95 degree 2 poles (-8.0806, -26.3341) (-7.6061, -26.3341) (-6.9338, -26.7346) (-6.741, -27.1696) knots 0 0 0 1 2 2 2
  spline S96 degree 2 poles (-6.741, -27.1696) (-6.563, -27.5551) (-6.4296, -28.6031) (-6.395, -29.2111) knots 0 0 0 1 2 2 2
  line L122 (-6.395, -29.2111) -> (-6.2467, -29.2111)
  spline S97 degree 2 poles (-6.2467, -29.2111) (-5.9797, -29.2111) (-5.6485, -29.048) (-5.5546, -28.8997) knots 0 0 0 1 2 2 2
  spline S98 degree 2 poles (-5.5546, -28.8997) (-5.4607, -28.7514) (-5.4014, -28.3263) (-5.4014, -28.0989) knots 0 0 0 1 2 2 2
  spline S99 degree 2 poles (-5.4014, -28.0989) (-5.4014, -27.832) (-5.5595, -27.1102) (-5.7128, -26.7494) knots 0 0 0 1 2 2 2
  line L123 (-5.7128, -26.7494) -> (-5.7128, -26.7049)
  line L124 (-5.7128, -26.7049) -> (-4.9268, -26.7049)
  spline S100 degree 2 poles (-4.9268, -26.7049) (-4.8675, -26.9175) (-4.7192, -27.7133) (-4.7192, -28.1038) knots 0 0 0 1 2 2 2
  spline S101 degree 2 poles (-4.7192, -28.1038) (-4.7192, -28.5784) (-4.8675, -29.226) (-5.0603, -29.483) knots 0 0 0 1 2 2 2
  spline S102 degree 2 poles (-5.0603, -29.483) (-5.2481, -29.7351) (-5.8462, -29.9823) (-6.2763, -29.9823) knots 0 0 0 1 2 2 2
  line L125 (-6.2763, -29.9823) -> (-9.4054, -29.9823)
  line L126 (-9.4054, -29.9823) -> (-9.4054, -29.2111)
  line L127 (-9.4054, -29.2111) -> (-8.921, -29.2111)
  line L128 (-8.2783, -29.2111) -> (-7.0079, -29.2111)
  spline S103 degree 2 poles (-7.0079, -29.2111) (-7.0326, -28.9343) (-7.1167, -28.0989) (-7.1958, -27.8369) knots 0 0 0 1 2 2 2
  spline S104 degree 2 poles (-7.1958, -27.8369) (-7.2897, -27.5304) (-7.6802, -27.13) (-8.0262, -27.13) knots 0 0 0 1 2 2 2
  spline S105 degree 2 poles (-8.0262, -27.13) (-8.4217, -27.13) (-8.8221, -27.5749) (-8.8221, -28) knots 0 0 0 1 2 2 2
  spline S106 degree 2 poles (-8.8221, -28) (-8.8221, -28.3609) (-8.5107, -28.9541) (-8.2783, -29.2111) knots 0 0 0 1 2 2 2
  line L129 (-9.4054, -34.6586) -> (-9.4054, -33.8875)
  line L130 (-9.4054, -33.8875) -> (-6.7954, -33.8875)
  spline S107 degree 2 poles (-6.7954, -33.8875) (-6.479, -33.8875) (-5.9352, -33.8282) (-5.7721, -33.7392) knots 0 0 0 1 2 2 2
  spline S108 degree 2 poles (-5.7721, -33.7392) (-5.5991, -33.6453) (-5.431, -33.3091) (-5.431, -33.0224) knots 0 0 0 1 2 2 2
  spline S109 degree 2 poles (-5.431, -33.0224) (-5.431, -32.7357) (-5.7375, -32.1277) (-5.9847, -31.836) knots 0 0 0 1 2 2 2
  line L131 (-5.9847, -31.836) -> (-9.4054, -31.836)
  line L132 (-9.4054, -31.836) -> (-9.4054, -31.0649)
  line L133 (-9.4054, -31.0649) -> (-4.8279, -31.0649)
  line L134 (-4.8279, -31.0649) -> (-4.8279, -31.836)
  line L135 (-4.8279, -31.836) -> (-5.3371, -31.836)
  spline S110 degree 2 poles (-5.3371, -31.836) (-5.0257, -32.182) (-4.6994, -32.8494) (-4.6994, -33.2251) knots 0 0 0 1 2 2 2
  spline S111 degree 2 poles (-4.6994, -33.2251) (-4.6994, -33.8974) (-5.5892, -34.6586) (-6.4345, -34.6586) knots 0 0 0 1 2 2 2
  line L136 (-6.4345, -34.6586) -> (-9.4054, -34.6586)
  spline S112 degree 2 poles (-9.4944, -37.1253) (-9.4944, -36.4975) (-8.7776, -35.7906) (-8.0015, -35.7906) knots 0 0 0 1 2 2 2
  line L137 (-8.0015, -35.7906) -> (-5.4656, -35.7906)
  line L138 (-5.4656, -35.7906) -> (-5.4656, -35.2716)
  line L139 (-5.4656, -35.2716) -> (-4.8279, -35.2716)
  line L140 (-4.8279, -35.2716) -> (-4.8279, -35.7906)
  line L141 (-4.8279, -35.7906) -> (-3.513, -35.7906)
  line L142 (-3.513, -35.7906) -> (-3.513, -36.5618)
  line L143 (-3.513, -36.5618) -> (-4.8279, -36.5618)
  line L144 (-4.8279, -36.5618) -> (-4.8279, -37.9805)
  line L145 (-4.8279, -37.9805) -> (-5.4656, -37.9805)
  line L146 (-5.4656, -37.9805) -> (-5.4656, -36.5618)
  line L147 (-5.4656, -36.5618) -> (-7.6456, -36.5618)
  spline S113 degree 2 poles (-7.6456, -36.5618) (-7.9916, -36.5618) (-8.3723, -36.5865) (-8.5354, -36.6705) knots 0 0 0 1 2 2 2
  spline S114 degree 2 poles (-8.5354, -36.6705) (-8.6787, -36.7397) (-8.8221, -37.0512) (-8.8221, -37.3181) knots 0 0 0 1 2 2 2
  spline S115 degree 2 poles (-8.8221, -37.3181) (-8.8221, -37.5059) (-8.7084, -37.8569) (-8.6738, -37.936) knots 0 0 0 1 2 2 2
  line L148 (-8.6738, -37.936) -> (-8.6738, -37.9805)
  line L149 (-8.6738, -37.9805) -> (-9.3659, -37.9805)
  spline S116 degree 2 poles (-9.3659, -37.9805) (-9.4252, -37.763) (-9.4944, -37.3181) (-9.4944, -37.1253) knots 0 0 0 1 2 2 2
  line L150 (-13.3766, 16.9437) -> (-15.7554, 17.5474)
  line L151 (-15.7554, 17.5474) -> (-15.7554, 17.9173)
  line L152 (-15.7554, 17.9173) -> (-13.9212, 18.4979)
  line L153 (-13.9212, 18.4979) -> (-15.7554, 19.0759)
  line L154 (-15.7554, 19.0759) -> (-15.7554, 19.4432)
  line L155 (-15.7554, 19.4432) -> (-13.3766, 20.0521)
  line L156 (-13.3766, 20.0521) -> (-13.3766, 19.6359)
  line L157 (-13.3766, 19.6359) -> (-15.2185, 19.2146)
  line L158 (-15.2185, 19.2146) -> (-13.3766, 18.652)
  line L159 (-13.3766, 18.652) -> (-13.3766, 18.3206)
  line L160 (-13.3766, 18.3206) -> (-15.2185, 17.7426)
  line L161 (-15.2185, 17.7426) -> (-13.3766, 17.347)
  line L162 (-13.3766, 17.347) -> (-13.3766, 16.9437)
  line L163 (-13.3766, 13.7095) -> (-15.7554, 14.3132)
  line L164 (-15.7554, 14.3132) -> (-15.7554, 14.6831)
  line L165 (-15.7554, 14.6831) -> (-13.9212, 15.2637)
  line L166 (-13.9212, 15.2637) -> (-15.7554, 15.8417)
  line L167 (-15.7554, 15.8417) -> (-15.7554, 16.209)
  line L168 (-15.7554, 16.209) -> (-13.3766, 16.8179)
  line L169 (-13.3766, 16.8179) -> (-13.3766, 16.4017)
  line L170 (-13.3766, 16.4017) -> (-15.2185, 15.9804)
  line L171 (-15.2185, 15.9804) -> (-13.3766, 15.4178)
  line L172 (-13.3766, 15.4178) -> (-13.3766, 15.0864)
  line L173 (-13.3766, 15.0864) -> (-15.2185, 14.5084)
  line L174 (-15.2185, 14.5084) -> (-13.3766, 14.1128)
  line L175 (-13.3766, 14.1128) -> (-13.3766, 13.7095)
  line L176 (-13.3766, 10.4753) -> (-15.7554, 11.079)
  line L177 (-15.7554, 11.079) -> (-15.7554, 11.4489)
  line L178 (-15.7554, 11.4489) -> (-13.9212, 12.0295)
  line L179 (-13.9212, 12.0295) -> (-15.7554, 12.6075)
  line L180 (-15.7554, 12.6075) -> (-15.7554, 12.9748)
  line L181 (-15.7554, 12.9748) -> (-13.3766, 13.5836)
  line L182 (-13.3766, 13.5836) -> (-13.3766, 13.1675)
  line L183 (-13.3766, 13.1675) -> (-15.2185, 12.7462)
  line L184 (-15.2185, 12.7462) -> (-13.3766, 12.1836)
  line L185 (-13.3766, 12.1836) -> (-13.3766, 11.8522)
  line L186 (-13.3766, 11.8522) -> (-15.2185, 11.2742)
  line L187 (-15.2185, 11.2742) -> (-13.3766, 10.8786)
  line L188 (-13.3766, 10.8786) -> (-13.3766, 10.4753)
  line L189 (-15.7554, 9.5017) -> (-15.7554, 10.0103)
  line L190 (-15.7554, 10.0103) -> (-15.1491, 10.0103)
  line L191 (-15.1491, 10.0103) -> (-15.1491, 9.5017)
  line L192 (-15.1491, 9.5017) -> (-15.7554, 9.5017)
  line L193 (-15.7554, 6.7504) -> (-15.7554, 8.9648)
  line L194 (-15.7554, 8.9648) -> (-15.3624, 8.9648)
  line L195 (-15.3624, 8.9648) -> (-12.9605, 7.2693)
  line L196 (-12.9605, 7.2693) -> (-12.9605, 8.8877)
  line L197 (-12.9605, 8.8877) -> (-12.5854, 8.8877)
  line L198 (-12.5854, 8.8877) -> (-12.5854, 6.7941)
  line L199 (-12.5854, 6.7941) -> (-12.9656, 6.7941)
  line L200 (-12.9656, 6.7941) -> (-15.3803, 8.5075)
  line L201 (-15.3803, 8.5075) -> (-15.3803, 6.7504)
  line L202 (-15.3803, 6.7504) -> (-15.7554, 6.7504)
  line L203 (-15.7554, 4.4975) -> (-15.7554, 4.8982)
  line L204 (-15.7554, 4.8982) -> (-14.399, 4.8982)
  spline S117 degree 2 poles (-14.399, 4.8982) (-14.2346, 4.8982) (-13.952, 4.9291) (-13.8673, 4.9753) knots 0 0 0 1 2 2 2
  spline S118 degree 2 poles (-13.8673, 4.9753) (-13.7774, 5.0241) (-13.69, 5.1988) (-13.69, 5.3478) knots 0 0 0 1 2 2 2
  spline S119 degree 2 poles (-13.69, 5.3478) (-13.69, 5.4968) (-13.8493, 5.8128) (-13.9777, 5.9643) knots 0 0 0 1 2 2 2
  line L205 (-13.9777, 5.9643) -> (-15.7554, 5.9643)
  line L206 (-15.7554, 5.9643) -> (-15.7554, 6.3651)
  line L207 (-15.7554, 6.3651) -> (-12.4441, 6.3651)
  line L208 (-12.4441, 6.3651) -> (-12.4441, 5.9643)
  line L209 (-12.4441, 5.9643) -> (-13.6412, 5.9643)
  spline S120 degree 2 poles (-13.6412, 5.9643) (-13.4794, 5.7845) (-13.3098, 5.4377) (-13.3098, 5.2425) knots 0 0 0 1 2 2 2
  spline S121 degree 2 poles (-13.3098, 5.2425) (-13.3098, 4.8931) (-13.7722, 4.4975) (-14.2115, 4.4975) knots 0 0 0 1 2 2 2
  line L210 (-14.2115, 4.4975) -> (-15.7554, 4.4975)
  line L211 (-15.7554, 3.5265) -> (-15.7554, 3.9272)
  line L212 (-15.7554, 3.9272) -> (-13.3766, 3.9272)
  line L213 (-13.3766, 3.9272) -> (-13.3766, 3.5265)
  line L214 (-13.3766, 3.5265) -> (-15.7554, 3.5265)
  line L215 (-12.981, 3.4982) -> (-12.981, 3.9529)
  line L216 (-12.981, 3.9529) -> (-12.5648, 3.9529)
  line L217 (-12.5648, 3.9529) -> (-12.5648, 3.4982)
  line L218 (-12.5648, 3.4982) -> (-12.981, 3.4982)
  line L219 (-15.7554, 2.1675) -> (-12.9605, 2.1675)
  line L220 (-12.9605, 2.1675) -> (-12.9605, 3.231)
  line L221 (-12.9605, 3.231) -> (-12.5854, 3.231)
  line L222 (-12.5854, 3.231) -> (-12.5854, 0.6827)
  line L223 (-12.5854, 0.6827) -> (-12.9605, 0.6827)
  line L224 (-12.9605, 0.6827) -> (-12.9605, 1.7462)
  line L225 (-12.9605, 1.7462) -> (-15.7554, 1.7462)
  line L226 (-15.7554, 1.7462) -> (-15.7554, 2.1675)
  spline S122 degree 2 poles (-15.8093, -0.6403) (-15.8093, -0.07) (-15.1697, 0.5568) (-14.5789, 0.5568) knots 0 0 0 1 2 2 2
  spline S123 degree 2 poles (-14.5789, 0.5568) (-13.9983, 0.5568) (-13.3098, -0.052) (-13.3098, -0.5427) knots 0 0 0 1 2 2 2
  spline S124 degree 2 poles (-13.3098, -0.5427) (-13.3098, -0.7636) (-13.4383, -1.1052) (-13.5744, -1.2311) knots 0 0 0 1 2 2 2
  spline S125 degree 2 poles (-13.5744, -1.2311) (-13.7106, -1.3596) (-14.1036, -1.4957) (-14.3888, -1.4957) knots 0 0 0 1 2 2 2
  line L227 (-14.3888, -1.4957) -> (-14.6071, -1.4957)
  line L228 (-14.6071, -1.4957) -> (-14.6071, 0.1509)
  spline S126 degree 2 poles (-14.6071, 0.1509) (-15.0207, 0.1509) (-15.46, -0.2652) (-15.46, -0.6351) knots 0 0 0 1 2 2 2
  spline S127 degree 2 poles (-15.46, -0.6351) (-15.46, -0.7661) (-15.4009, -1.0205) (-15.3547, -1.1232) knots 0 0 0 1 2 2 2
  spline S128 degree 2 poles (-15.3547, -1.1232) (-15.3033, -1.2311) (-15.2134, -1.3801) (-15.1723, -1.4289) knots 0 0 0 1 2 2 2
  line L229 (-15.1723, -1.4289) -> (-15.1723, -1.452)
  line L230 (-15.1723, -1.452) -> (-15.609, -1.452)
  spline S129 degree 2 poles (-15.609, -1.452) (-15.6372, -1.3827) (-15.7194, -1.172) (-15.7426, -1.0898) knots 0 0 0 1 2 2 2
  spline S130 degree 2 poles (-15.7426, -1.0898) (-15.776, -0.9742) (-15.8093, -0.7841) (-15.8093, -0.6403) knots 0 0 0 1 2 2 2
  spline S131 degree 2 poles (-14.3014, -1.1052) (-14.1396, -1.1001) (-13.9032, -1.0333) (-13.8236, -0.9691) knots 0 0 0 1 2 2 2
  spline S132 degree 2 poles (-13.8236, -0.9691) (-13.7337, -0.8997) (-13.6386, -0.6814) (-13.6386, -0.5195) knots 0 0 0 1 2 2 2
  spline S133 degree 2 poles (-13.6386, -0.5195) (-13.6386, -0.3603) (-13.7337, -0.1368) (-13.8262, -0.0443) knots 0 0 0 1 2 2 2
  spline S134 degree 2 poles (-13.8262, -0.0443) (-13.9212, 0.0456) (-14.1498, 0.1381) (-14.3014, 0.1509) knots 0 0 0 1 2 2 2
  line L231 (-14.3014, 0.1509) -> (-14.3014, -1.1052)
  spline S135 degree 2 poles (-15.8093, -2.8469) (-15.8093, -2.6003) (-15.6578, -2.1919) (-15.5036, -2.0454) knots 0 0 0 1 2 2 2
  spline S136 degree 2 poles (-15.5036, -2.0454) (-15.3521, -1.899) (-14.8845, -1.7372) (-14.5711, -1.7372) knots 0 0 0 1 2 2 2
  spline S137 degree 2 poles (-14.5711, -1.7372) (-14.2577, -1.7372) (-13.8005, -1.9042) (-13.6463, -2.0454) knots 0 0 0 1 2 2 2
  spline S138 degree 2 poles (-13.6463, -2.0454) (-13.4896, -2.1867) (-13.3227, -2.6055) (-13.3227, -2.8469) knots 0 0 0 1 2 2 2
  spline S139 degree 2 poles (-13.3227, -2.8469) (-13.3227, -3.0422) (-13.4331, -3.407) (-13.5051, -3.5482) knots 0 0 0 1 2 2 2
  line L232 (-13.5051, -3.5482) -> (-13.9546, -3.5482)
  line L233 (-13.9546, -3.5482) -> (-13.9546, -3.5251)
  spline S140 degree 2 poles (-13.9546, -3.5251) (-13.9186, -3.4815) (-13.8262, -3.3479) (-13.7774, -3.2528) knots 0 0 0 1 2 2 2
  spline S141 degree 2 poles (-13.7774, -3.2528) (-13.7363, -3.168) (-13.672, -2.942) (-13.672, -2.8392) knots 0 0 0 1 2 2 2
  spline S142 degree 2 poles (-13.672, -2.8392) (-13.672, -2.5284) (-14.1421, -2.1508) (-14.5711, -2.1508) knots 0 0 0 1 2 2 2
  spline S143 degree 2 poles (-14.5711, -2.1508) (-14.9899, -2.1508) (-15.46, -2.5156) (-15.46, -2.8392) knots 0 0 0 1 2 2 2
  spline S144 degree 2 poles (-15.46, -2.8392) (-15.46, -3.0345) (-15.2981, -3.389) (-15.1723, -3.5251) knots 0 0 0 1 2 2 2
  line L234 (-15.1723, -3.5251) -> (-15.1723, -3.5482)
  line L235 (-15.1723, -3.5482) -> (-15.6218, -3.5482)
  spline S145 degree 2 poles (-15.6218, -3.5482) (-15.6501, -3.4892) (-15.7297, -3.3093) (-15.7477, -3.2374) knots 0 0 0 1 2 2 2
  spline S146 degree 2 poles (-15.7477, -3.2374) (-15.7785, -3.1347) (-15.8093, -2.9728) (-15.8093, -2.8469) knots 0 0 0 1 2 2 2
  line L236 (-15.7554, -5.7806) -> (-15.7554, -5.3799)
  line L237 (-15.7554, -5.3799) -> (-14.399, -5.3799)
  spline S147 degree 2 poles (-14.399, -5.3799) (-14.2346, -5.3799) (-13.952, -5.349) (-13.8673, -5.3028) knots 0 0 0 1 2 2 2
  spline S148 degree 2 poles (-13.8673, -5.3028) (-13.7774, -5.254) (-13.69, -5.0793) (-13.69, -4.9303) knots 0 0 0 1 2 2 2
  spline S149 degree 2 poles (-13.69, -4.9303) (-13.69, -4.7813) (-13.8493, -4.4653) (-13.9777, -4.3138) knots 0 0 0 1 2 2 2
  line L238 (-13.9777, -4.3138) -> (-15.7554, -4.3138)
  line L239 (-15.7554, -4.3138) -> (-15.7554, -3.913)
  line L240 (-15.7554, -3.913) -> (-12.4441, -3.913)
  line L241 (-12.4441, -3.913) -> (-12.4441, -4.3138)
  line L242 (-12.4441, -4.3138) -> (-13.6412, -4.3138)
  spline S150 degree 2 poles (-13.6412, -4.3138) (-13.4794, -4.4936) (-13.3098, -4.8404) (-13.3098, -5.0356) knots 0 0 0 1 2 2 2
  spline S151 degree 2 poles (-13.3098, -5.0356) (-13.3098, -5.385) (-13.7722, -5.7806) (-14.2115, -5.7806) knots 0 0 0 1 2 2 2
  line L243 (-14.2115, -5.7806) -> (-15.7554, -5.7806)
  line L244 (-15.7554, -6.0324) -> (-12.5854, -7.101)
  line L245 (-12.5854, -7.101) -> (-12.5854, -7.6199)
  line L246 (-12.5854, -7.6199) -> (-15.7554, -8.6886)
  line L247 (-15.7554, -8.6886) -> (-15.7554, -8.2442)
  line L248 (-15.7554, -8.2442) -> (-14.8691, -7.9564)
  line L249 (-14.8691, -7.9564) -> (-14.8691, -6.7465)
  line L250 (-14.8691, -6.7465) -> (-15.7554, -6.4588)
  line L251 (-15.7554, -6.4588) -> (-15.7554, -6.0324)
  line L252 (-14.5095, -7.8408) -> (-13.017, -7.3502)
  line L253 (-13.017, -7.3502) -> (-14.5095, -6.8621)
  line L254 (-14.5095, -6.8621) -> (-14.5095, -7.8408)
  line L255 (-15.7554, -10.0938) -> (-15.7554, -8.8658)
  line L256 (-15.7554, -8.8658) -> (-15.4317, -8.8658)
  line L257 (-15.4317, -8.8658) -> (-15.4317, -9.2691)
  line L258 (-15.4317, -9.2691) -> (-12.9091, -9.2691)
  line L259 (-12.9091, -9.2691) -> (-12.9091, -8.8658)
  line L260 (-12.9091, -8.8658) -> (-12.5854, -8.8658)
  line L261 (-12.5854, -8.8658) -> (-12.5854, -10.0938)
  line L262 (-12.5854, -10.0938) -> (-12.9091, -10.0938)
  line L263 (-12.9091, -10.0938) -> (-12.9091, -9.6904)
  line L264 (-12.9091, -9.6904) -> (-15.4317, -9.6904)
  line L265 (-15.4317, -9.6904) -> (-15.4317, -10.0938)
  line L266 (-15.4317, -10.0938) -> (-15.7554, -10.0938)
  line L267 (-15.7554, -11.2061) -> (-15.7554, -10.6974)
  line L268 (-15.7554, -10.6974) -> (-15.1491, -10.6974)
  line L269 (-15.1491, -10.6974) -> (-15.1491, -11.2061)
  line L270 (-15.1491, -11.2061) -> (-15.7554, -11.2061)
  spline S152 degree 2 poles (-15.8119, -13.1738) (-15.8119, -12.8656) (-15.6038, -12.3441) (-15.3958, -12.154) knots 0 0 0 1 2 2 2
  spline S153 degree 2 poles (-15.3958, -12.154) (-15.1902, -11.9639) (-14.5737, -11.7558) (-14.173, -11.7558) knots 0 0 0 1 2 2 2
  spline S154 degree 2 poles (-14.173, -11.7558) (-13.7748, -11.7558) (-13.1839, -11.9588) (-12.9656, -12.1514) knots 0 0 0 1 2 2 2
  spline S155 degree 2 poles (-12.9656, -12.1514) (-12.7524, -12.3415) (-12.5289, -12.8604) (-12.5289, -13.1815) knots 0 0 0 1 2 2 2
  spline S156 degree 2 poles (-12.5289, -13.1815) (-12.5289, -13.3408) (-12.5751, -13.6208) (-12.6111, -13.739) knots 0 0 0 1 2 2 2
  spline S157 degree 2 poles (-12.6111, -13.739) (-12.6445, -13.8418) (-12.7395, -14.055) (-12.796, -14.1603) knots 0 0 0 1 2 2 2
  line L271 (-12.796, -14.1603) -> (-13.3047, -14.1603)
  line L272 (-13.3047, -14.1603) -> (-13.3047, -14.1269)
  spline S158 degree 2 poles (-13.3047, -14.1269) (-13.2533, -14.0704) (-13.1095, -13.8957) (-13.0401, -13.7698) knots 0 0 0 1 2 2 2